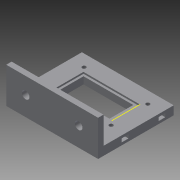
# Autodesk Inventor part: SampleBase
Saved by Autodesk Inventor 2015 (Build 190159000, 159)
## iProperties
Created: 2014-06-06
Part Number: SampleBase
Material: Generic
Document SubType Name: Modeling
Designer: miles90
Density: 1 g/cm^3
Appearance: Default
Author: miles90
Autodesk Inventor part; units mm, degrees
ref_plane "YZ Plane" through (0, 0, 0) normal (1, 0, 0) x (0, 1, 0)
ref_plane "XZ Plane" through (0, 0, 0) normal (0, 1, 0) x (-1, 0, 0)
ref_plane "XY Plane" through (0, 0, 0) normal (0, 0, 1) x (1, 0, 0)
sketch "Sketch1" plane through (0, 0, 0) normal (0, 1, 0) x (-1, 0, 0)
  line L0 (52.3087, -21.6726) -> (-32.6913, -21.6726)
  line L1 (-32.6913, -21.6726) -> (-32.6913, 48.3274)
  line L2 (-32.6913, 48.3274) -> (52.3087, 48.3274)
  line L3 (52.3087, 48.3274) -> (52.3087, -21.6726)
  dimension "d4" = 70
  dimension "d5" = 85
  constraints: 8 end point, 2 parallel, 1 horizontal, 1 perpendicular
  measures "d4" distance of L2.end L0.start
  measures "d5" distance of L0.start L0.end
extrude "Extrusion1" add sketch "Sketch1" along normal blind 33
sketch "Sketch2" plane through (0, 33, 0) normal (0, 1, 0) x (1, 0, 0)
  line L0 (32.6913, 21.6726) -> (-52.3087, 21.6726) projected
  line L1 (-52.3087, 21.6726) -> (-52.3087, -48.3274) projected
  line L2 (-52.3087, -48.3274) -> (32.6913, -48.3274) projected
  line L3 (32.6913, -48.3274) -> (32.6913, 21.6726) projected
  line L4 (-52.3087, 21.6726) -> (32.6913, 21.6726)
  line L5 (32.6913, 21.6726) -> (32.6913, -43.3274)
  line L6 (32.6913, -43.3274) -> (-52.3087, -43.3274)
  line L7 (-52.3087, -43.3274) -> (-52.3087, 21.6726)
  point P0 (0, 0)
  dimension "d8" = 0
  dimension "d9" = 0
  dimension "d10" = 5
  constraints: 8 end point, 1 collinear, 1 parallel, 1 perpendicular
  measures "d8" distance between parallel lines of L1 L7
  measures "d9" distance between parallel lines of L5 L3
  measures "d10" distance between parallel lines of L6 L2
extrude "Extrusion2" cut sketch "Sketch2" against normal blind 25 contours L3 L6 L1 L0
sketch "Sketch3" plane through (0, 8, 0) normal (0, 1, 0) x (1, 0, 0)
  line L0 (32.6913, -43.3274) -> (-52.3087, -43.3274) projected
  line L1 (-35.8087, 6.6726) -> (16.1913, 6.6726)
  line L2 (16.1913, 6.6726) -> (16.1913, -19.3274)
  line L3 (16.1913, -19.3274) -> (-35.8087, -19.3274)
  line L4 (-35.8087, -19.3274) -> (-35.8087, 6.6726)
  line L5 (-52.3087, 21.6726) -> (32.6913, 21.6726)
  line L6 (-52.3087, -48.3274) -> (-52.3087, 21.6726) projected
  line L7 (-9.8087, -43.3274) -> (-9.8087, 21.6726) construction
  circle A0 centre (-39.3087, -23.3274) radius 1.75
  circle A1 centre (-39.3087, 10.6726) radius 1.75
  circle A2 centre (19.6913, 10.6726) radius 1.75
  circle A3 centre (19.6913, -23.3274) radius 1.75
  line L8 (-52.6639, -6.3274) -> (32.3361, -6.3274) construction
  point P0 (0, 0)
  dimension "d106" = 26
  dimension "d107" = 3.5
  dimension "d110" = 34
  dimension "d111" = 59
  dimension "d144" = 52
  dimension "d145" = 15
  constraints: 14 end point, 4 centre point, 4 perpendicular, 3 equal radius, 3 symmetric about line, 2 midpoint, 2 parallel, 1 horizontal, 2 other
  measures "d106" distance between parallel lines of L1 L3
  measures "d107" diameter of A0
  measures "d110" distance of A1.centre A0.centre
  measures "d111" distance of A0.centre A3.centre
  measures "d144" distance of L1.start L1.end
  measures "d145" distance between parallel lines of L5 L1
extrude "Extrusion3" cut sketch "Sketch3" against normal blind 1.5
sketch "Sketch4" plane through (0, 6.5, 0) normal (0, 1, 0) x (1, 0, 0)
  line L0 (-35.8087, 6.6726) -> (16.1913, 6.6726) projected
  line L1 (-35.8087, -19.3274) -> (-35.8087, 6.6726) projected
  line L2 (16.1913, -19.3274) -> (-35.8087, -19.3274) projected
  line L3 (16.1913, 6.6726) -> (16.1913, -19.3274) projected
  line L4 (-33.8087, 4.6726) -> (12.1913, 4.6726)
  line L5 (12.1913, 4.6726) -> (12.1913, -17.3274)
  line L6 (12.1913, -17.3274) -> (-33.8087, -17.3274)
  line L7 (-33.8087, -17.3274) -> (-33.8087, 4.6726)
  point P0 (0, 0)
  dimension "d20" = 2
  dimension "d21" = 2
  dimension "d22" = 2
  dimension "d23" = 4
  constraints: 8 end point, 2 parallel, 1 horizontal, 1 perpendicular
  measures "d20" distance between parallel lines of L1 L7
  measures "d21" distance between parallel lines of L0 L4
  measures "d22" distance between parallel lines of L2 L6
  measures "d23" distance between parallel lines of L3 L5
extrude "Extrusion4" cut sketch "Sketch4" against normal blind 1 contours L4 L5 L6 L7
sketch "Sketch10" plane through (32.6913, 8, 43.3274) normal (0, 0, -1) x (-1, 0, 0)
  line L0 (85, 25) -> (85, 0) projected
  line L1 (0, 25) -> (85, 25) projected
  circle A0 centre (18, 9.75) radius 3.5
  circle A1 centre (67, 9.75) radius 3.5
  point P0 (32.6913, -8)
  dimension "d53" = 15.25
  dimension "d55" = 15.25
  dimension "d58" = 7
  dimension "d59" = 7
  dimension "d70" = 49
  dimension "d71" = 18
  constraints: 2 centre point
  measures "d53" distance from line of L1 A1.centre
  measures "d55" distance from line of L1 A0.centre
  measures "d58" diameter of A0
  measures "d59" diameter of A1
  measures "d70" distance of A1.centre A0.centre
  measures "d71" distance from line of L0 A1.centre
extrude "Extrusion9" cut sketch "Sketch10" against normal blind 5
sketch "Sketch16" plane through (16.1913, 8, -6.6726) normal (-1, 0, 0) x (0, 0, 1)
  line L0 (0, 0) -> (26, 0) projected
  line L1 (0, 0) -> (0, -1.5) projected
  line L2 (0, -1.5) -> (26, -1.5) projected
  line L3 (26, 0) -> (26, -1.5) projected
  point P0 (6.6726, -8)
sketch "Sketch17" plane through (0, 5.5, 0) normal (0, 1, 0) x (1, 0, 0)
  line L0 (-33.8087, 4.6726) -> (12.1913, 4.6726) projected
  line L1 (-33.8087, -17.3274) -> (-33.8087, 4.6726) projected
  line L2 (12.1913, -17.3274) -> (-33.8087, -17.3274) projected
  line L3 (12.1913, 4.6726) -> (12.1913, -17.3274) projected
  line L4 (-33.8087, 4.6726) -> (12.1913, 4.6726)
  line L5 (12.1913, 4.6726) -> (12.1913, -17.3274)
  line L6 (12.1913, -17.3274) -> (-33.8087, -17.3274)
  line L7 (-33.8087, -17.3274) -> (-33.8087, 4.6726)
  point P0 (0, 0)
  dimension "d93" = 0
  dimension "d94" = 0
  dimension "d95" = 0
  dimension "d96" = 0
  constraints: 8 end point, 2 parallel, 1 horizontal, 1 perpendicular
  measures "d93" distance between parallel lines of L0 L4
  measures "d94" distance between parallel lines of L3 L5
  measures "d95" distance between parallel lines of L1 L7
  measures "d96" distance between parallel lines of L2 L6
extrude "Extrusion14" cut sketch "Sketch17" along normal through all both and the other way through all
sketch "Sketch20" plane through (32.6913, 0, 48.3274) normal (1, 0, 0) x (0, 0, -1)
  line L0 (21.875, 5.625) -> (28.125, 5.625)
  line L1 (28.125, 5.625) -> (28.125, 2.375)
  line L2 (28.125, 2.375) -> (21.875, 2.375)
  line L3 (21.875, 2.375) -> (21.875, 5.625)
  line L4 (55.875, 5.625) -> (62.125, 5.625)
  line L5 (62.125, 5.625) -> (62.125, 2.375)
  line L6 (62.125, 2.375) -> (55.875, 2.375)
  line L7 (55.875, 2.375) -> (55.875, 5.625)
  line L8 (25, 6.5) -> (25, 2.375) construction
  line L9 (59, 6.5) -> (59, 2.375) construction
  line L10 (23.25, 6.5) -> (26.75, 6.5) construction
  line L11 (57.25, 6.5) -> (60.75, 6.5) construction
  line L12 (70, 0) -> (70, 8) construction
  line L13 (70, 4) -> (0, 4) construction
  line L14 (0, 0) -> (0, 33) construction
  point P0 (48.3274, 0)
  dimension "d113" = 3.25
  dimension "d125" = 6.25
  constraints: 22 end point, 5 midpoint, 4 parallel, 2 equal length, 2 horizontal, 2 perpendicular, 2 vertical, 1 collinear, 1 point on line, 1 other
  measures "d113" distance of L0.end L1.end
  measures "d125" distance between parallel lines of L1 L3
extrude "Extrusion16" cut sketch "Sketch20" against normal blind 16
sketch "Sketch21" plane through (-52.3087, 0, -21.6726) normal (-1, 0, 0) x (0, 0, 1)
  line L0 (7.875, 5.625) -> (14.125, 5.625)
  line L1 (14.125, 5.625) -> (14.125, 2.375)
  line L2 (14.125, 2.375) -> (7.875, 2.375)
  line L3 (7.875, 2.375) -> (7.875, 5.625)
  line L4 (41.875, 5.625) -> (48.125, 5.625)
  line L5 (48.125, 5.625) -> (48.125, 2.375)
  line L6 (48.125, 2.375) -> (41.875, 2.375)
  line L7 (41.875, 2.375) -> (41.875, 5.625)
  line L8 (7.875, 2.375) -> (14.125, 2.375) projected
  line L9 (41.875, 2.375) -> (48.125, 2.375) projected
  line L10 (48.125, 5.625) -> (41.875, 5.625) projected
  line L11 (41.875, 5.625) -> (41.875, 2.375) projected
  line L12 (48.125, 2.375) -> (48.125, 5.625) projected
  line L13 (14.125, 2.375) -> (14.125, 5.625) projected
  line L14 (7.875, 5.625) -> (7.875, 2.375) projected
  line L15 (14.125, 5.625) -> (7.875, 5.625) projected
  constraints: 16 end point, 8 collinear, 4 parallel, 2 horizontal, 2 perpendicular
extrude "Extrusion17" cut sketch "Sketch21" against normal blind 16
sketch "Sketch22" plane through (0, 8, 0) normal (0, 1, 0) x (1, 0, 0)
  circle A0 centre (-39.3087, -23.3274) radius 1.75
  circle A1 centre (19.6913, 10.6726) radius 1.75 projected
  circle A2 centre (-39.3087, 10.6726) radius 1.75
  circle A3 centre (19.6913, -23.3274) radius 1.75
  circle A4 centre (19.6913, 10.6726) radius 1.75
  circle A5 centre (19.6913, -23.3274) radius 1.75 projected
  circle A6 centre (-39.3087, 10.6726) radius 1.75 projected
  circle A7 centre (-39.3087, -23.3274) radius 1.75 projected
  point P0 (0, 0)
  constraints: 4 centre point, 4 concentric, 4 equal radius
extrude "Extrusion18" cut sketch "Sketch22" against normal through all
body "Solid1"
